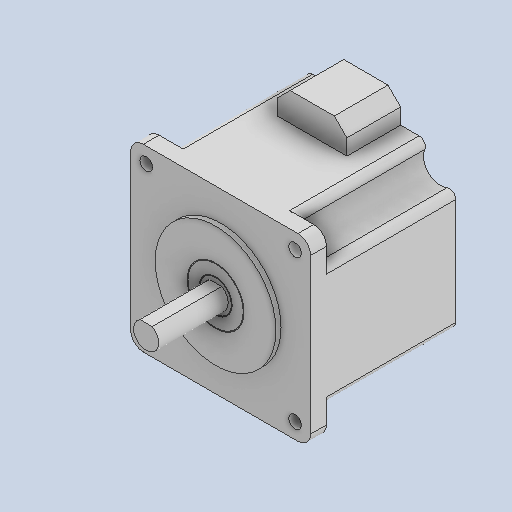
# Autodesk Inventor part: SouluckNema23-0.7N-24V
Saved by Autodesk Inventor 2025.2 (Build 292293000, 293)
## iProperties
Created: 2025-02-08
Part Number: SouluckNema23-0.7N-24V
Material: Generic
Document SubType Name: Modeling
Designer: LattePanda
Density: 1 g/cm^3
Appearance: Default
Author: LattePanda
Autodesk Inventor part; units mm, degrees
ref_plane "YZ Plane" through (0, 0, 0) normal (1, 0, 0) x (0, 1, 0)
ref_plane "XZ Plane" through (0, 0, 0) normal (0, 1, 0) x (-1, 0, 0)
ref_plane "XY Plane" through (0, 0, 0) normal (0, 0, 1) x (1, 0, 0)
sketch "Sketch1" plane through (0, 0, 0) normal (0, 0, 1) x (1, 0, 0)
  line L0 (-28.5, 28.5) -> (28.5, 28.5)
  line L1 (28.5, 28.5) -> (28.5, -28.5)
  line L2 (28.5, -28.5) -> (-28.5, -28.5)
  line L3 (-28.5, -28.5) -> (-28.5, 28.5)
  line L4 (-28.5, 28.5) -> (28.5, -28.5) construction
  line L5 (28.5, 28.5) -> (-28.5, -28.5) construction
  line L6 (-23.57, 23.57) -> (23.57, 23.57) construction
  circle A0 centre (-23.57, 23.57) radius 2
  line L7 (0, 0) -> (0, 28.5) construction
  line L8 (-28.5, 0) -> (28.5, 0) construction
  circle A1 centre (23.57, 23.57) radius 2
  circle A2 centre (-23.57, -23.57) radius 2
  circle A3 centre (23.57, -23.57) radius 2
  dimension "d0" = 57
  dimension "d1" = 47.14
  dimension "d2" = 4
  constraints: 18 end point, 5 midpoint, 4 centre point, 3 symmetric about line, 2 horizontal, 2 parallel, 2 perpendicular, 2 point on line, 1 coincident, 3 other
  measures "d0" distance of L0.start L0.end
  measures "d1" distance of L6.start L6.end
  measures "d2" diameter of A0
extrude "Extrusion1" add sketch "Sketch1" against normal blind 5
fillet "Fillet1" radius 4 4 edges at (28.5, -28.5, -2.5) (28.5, 28.5, -2.5) (-28.5, 28.5, -2.5) (-28.5, -28.5, -2.5)
sketch "Sketch2" plane through (0, 0, 0) normal (0, 0, 1) x (1, 0, 0)
  circle A0 centre (0, 0) radius 19.125
  dimension "d6" = 38.25
  constraints: 1 centre point, 1 coincident
  measures "d6" diameter of A0
extrude "Extrusion2" add sketch "Sketch2" along normal blind 1.6
sketch "Sketch3" plane through (0, 0, 1.6) normal (0, 0, 1) x (1, 0, 0)
  circle A0 centre (0, 0) radius 9
  circle A1 centre (0, 0) radius 5
  circle A2 centre (0, 0) radius 8.75
  circle A3 centre (0, 0) radius 5.25
  dimension "d9" = 18
  dimension "d10" = 4
  dimension "d11" = 0.25
  dimension "d12" = 0.25
  constraints: 4 centre point, 2 coincident
  measures "d9" diameter of A0
  measures "d10" radial gap between concentric circles of A0 A1
  measures "d11" radial gap between concentric circles of A0 A2
  measures "d12" radial gap between concentric circles of A1 A3
extrude "Extrusion3" cut sketch "Sketch3" against normal blind 0.25
sketch "Sketch4" plane through (0, 0, 1.6) normal (0, 0, 1) x (1, 0, 0)
  circle A0 centre (0, 0) radius 4
  dimension "d15" = 8
  constraints: 1 centre point, 1 coincident
  measures "d15" diameter of A0
extrude "Extrusion4" add sketch "Sketch4" along normal blind 22
sketch "Sketch5" plane through (0, 0, 23.6) normal (0, 0, 1) x (1, 0, 0)
  circle A0 centre (0, 0) radius 4 projected
  line L0 (-1.9365, 3.5) -> (1.9365, 3.5)
  line L1 (0, -4) -> (0, 3.5) construction
  dimension "d18" = 7.5
  constraints: 4 end point, 3 point on circle, 1 horizontal, 1 midpoint
  measures "d18" distance of L1.start L1.end
extrude "Extrusion5" cut sketch "Sketch5" against normal up to surface (22 mm away) contours L0 A0 picked at (-0.3981, 3.6058)
sketch "Sketch6" plane through (0, 0, -5) normal (0, 0, -1) x (-1, 0, 0)
  arc A0 (24.5, -28.5) -> (28.5, -24.5) centre (24.5, -24.5) ccw projected
  line L0 (28.5, -24.5) -> (28.5, 24.5) projected
  arc A1 (28.5, 24.5) -> (24.5, 28.5) centre (24.5, 24.5) ccw projected
  line L1 (24.5, 28.5) -> (-24.5, 28.5) projected
  arc A2 (-24.5, 28.5) -> (-28.5, 24.5) centre (-24.5, 24.5) ccw projected
  line L2 (-28.5, 24.5) -> (-28.5, -24.5) projected
  arc A3 (-28.5, -24.5) -> (-24.5, -28.5) centre (-24.5, -24.5) ccw projected
  line L3 (-24.5, -28.5) -> (24.5, -28.5) projected
  circle A4 centre (-23.57, -23.57) radius 2 projected
  circle A5 centre (23.57, -23.57) radius 2 projected
  circle A6 centre (-23.57, 23.57) radius 2 projected
  circle A7 centre (23.57, 23.57) radius 2 projected
  circle A8 centre (23.57, 23.57) radius 5.3152
  line L4 (0, 28.5) -> (0, -28.5)
  line L5 (28.5, 0) -> (-28.5, 0)
  circle A9 centre (23.57, -23.57) radius 5.3152
  circle A10 centre (-23.57, 23.57) radius 5.3152
  circle A11 centre (-23.57, -23.57) radius 5.3152
  point P0 (0, 0)
  point P1 (28.5, 21.5834)
  point P2 (21.5834, 28.5)
  point P3 (-21.5834, 28.5)
  point P4 (-28.5, 21.5834)
  point P5 (-28.5, -21.5834)
  point P6 (-21.5834, -28.5)
  point P7 (21.5834, -28.5)
  point P8 (28.5, -21.5834)
  constraints: 4 centre point, 4 end point, 4 midpoint, 3 symmetric about line, 1 coincident, 3 other
extrude "Extrusion6" add sketch "Sketch6" along normal blind 41 contours L3 L4 L5 L0 A9 | L3 A11 L2 L5 L4 | L5 L2 A10 L1 L4 | L4 L1 A8 L0 L5
fillet "Fillet2" radius 2 8 edges at (-28.5, 21.5834, -25.5) (-21.5834, 28.5, -25.5) (-28.5, -21.5834, -25.5) (-21.5834, -28.5, -25.5) (21.5834, 28.5, -25.5) (28.5, 21.5834, -25.5) (28.5, -21.5834, -25.5) (21.5834, -28.5, -25.5)
sketch "Sketch8" plane through (-24.5, 28.5, 0) normal (0, 1, 0) x (1, 0, 0)
  line L0 (41.3672, 46) -> (7.6328, 46) projected
  line L1 (35.5, 46) -> (13.5, 46)
  line L2 (13.5, 46) -> (13.5, 29)
  line L3 (13.5, 29) -> (35.5, 29)
  line L4 (35.5, 29) -> (35.5, 46)
  line L5 (24.5, 0) -> (24.5, 46) construction
  point P0 (24.5, 29)
  point P1 (13.5, 46)
  dimension "d24" = 22
  dimension "d25" = 17
  constraints: 10 end point, 2 midpoint, 2 parallel, 2 perpendicular, 2 point on line, 1 horizontal
  measures "d24" distance of L2.end L3.end
  measures "d25" distance of L1.end L2.end
extrude "Extrusion7" add sketch "Sketch8" along normal blind 9
chamfer "Chamfer1" distance 4 angle 45 2 edges at (11, 37.5, -37.5) (-11, 37.5, -37.5)
body "Solid1"
